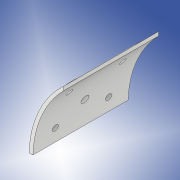
# Autodesk Inventor part: SJ009
Saved by Autodesk Inventor 2017 SP1 (Build 210196100, 196)
## iProperties
Created: 2017-06-10
Part Number: SJ009
Material: ABS Plastic
Document SubType Name: Modeling
Designer: Zach
Density: 1.06 g/cm^3
Appearance: CR White
Author: Zach
Autodesk Inventor part; units mm, degrees
ref_plane "YZ Plane" through (0, 0, 0) normal (1, 0, 0) x (0, 1, 0)
sketch "Sketch1" plane through (0, 0, 0) normal (0, 0, 1) x (1, 0, 0)
  arc A0 (45, 98) -> (0, 0) centre (139.9137, -4.9145) ccw
  line L0 (45, 98) -> (45, 93)
  line L1 (0, 0) -> (5, 0)
  arc A1 (45, 93) -> (5, 0) centre (144.908, -5.0734) ccw
  dimension "d0" = 140
  dimension "d1" = 98
  dimension "d3" = 45
  dimension "d4" = 5
  dimension "d5" = 5
  dimension "d6" = 140
  constraints: 4 end point, 4 point on circle, 2 centre point, 1 horizontal, 1 vertical
  measures "d0" radius of A0
  measures "d1" vertical distance of L1.start L0.start
  measures "d3" horizontal distance of L1.start L0.start
  measures "d4" distance of L0.start L0.end
  measures "d5" distance of L1.start L1.end
  measures "d6" radius of A1
extrude "Extrusion1" add sketch "Sketch1" along normal blind 125
ref_plane "Work Plane1" through (0, 0, 62.5) normal (0, 0, -1) x (-1, 0, 0)
sketch "Sketch3" plane through (0, 0, 62.5) normal (0, 0, -1) x (-1, 0, 0)
  arc A0 (0, 0) -> (-45, 98) centre (-139.9137, -4.9145) ccw projected
  line L0 (0, 0) -> (10, 0)
  arc A1 (10, 0) -> (-45, 98) centre (-152.788, -26.9269) ccw
  arc A2 (0, 0) -> (-45, 98) centre (-139.9137, -4.9145) ccw
  dimension "d19" = 10
  dimension "d20" = 165
  constraints: 4 point on circle, 2 centre point, 2 end point, 1 concentric, 1 horizontal
  measures "d19" distance of L0.start L0.end
  measures "d20" radius of A1
extrude "Extrusion3" add sketch "Sketch3" along normal mid plane 85
ref_plane "Work Plane2" through (-10, 0, 62.5) normal (-0.9866, 0.1632, 0) x (-0.1632, -0.9866, 0)
sketch "Sketch2" plane through (-10, 0, 62.5) normal (-0.9866, 0.1632, 0) x (-0.1632, -0.9866, 0)
  circle A0 centre (-20.6619, -35) radius 4
  circle A1 centre (-72.6619, -35) radius 4
  circle A2 centre (-20.6619, 35) radius 4
  circle A3 centre (-72.6619, 35) radius 4
  line L0 (0, 42.5) -> (0, -42.5) projected
  line L1 (-72.6619, 35) -> (-20.6619, 35) construction
  line L2 (-20.6619, 35) -> (-20.6619, -35) construction
  line L3 (-20.6619, -35) -> (-72.6619, -35) construction
  line L4 (-72.6619, -35) -> (-72.6619, 35) construction
  line L5 (-105.6619, -42.5) -> (-105.6619, 42.5) projected
  point P0 (0, 0)
  point P1 (-20.6619, 0)
  point P2 (0, 0)
  dimension "d9" = 8
  dimension "d10" = 8
  dimension "d12" = 52
  dimension "d14" = 8
  dimension "d15" = 8
  dimension "d16" = 70
  dimension "d23" = 33
  constraints: 8 end point, 4 centre point, 3 horizontal alignment, 2 midpoint, 2 parallel, 2 vertical alignment, 1 horizontal, 1 perpendicular
  measures "d9" diameter of A0
  measures "d10" diameter of A1
  measures "d12" distance of A1.centre L2.end
  measures "d14" diameter of A2
  measures "d15" diameter of A3
  measures "d16" distance of A2.centre L2.end
  measures "d23" distance from line of L5 A1.centre
extrude "Extrusion2" cut sketch "Sketch2" against normal through all
sketch "Sketch4" plane through (-10, 0, 62.5) normal (-0.9866, 0.1632, 0) x (-0.1632, -0.9866, 0)
  circle A0 centre (-38, 0) radius 5
  line L0 (0, 42.5) -> (0, -42.5) projected
  point P0 (-1.6319, -62.5)
  point P1 (0, 0)
  dimension "d24" = 10
  dimension "d25" = 38
  constraints: 1 centre point, 1 horizontal alignment, 1 midpoint
  measures "d24" diameter of A0
  measures "d25" distance from line of L0 A0.centre
extrude "Extrusion4" cut sketch "Sketch4" against normal through all
body "Solid1"
